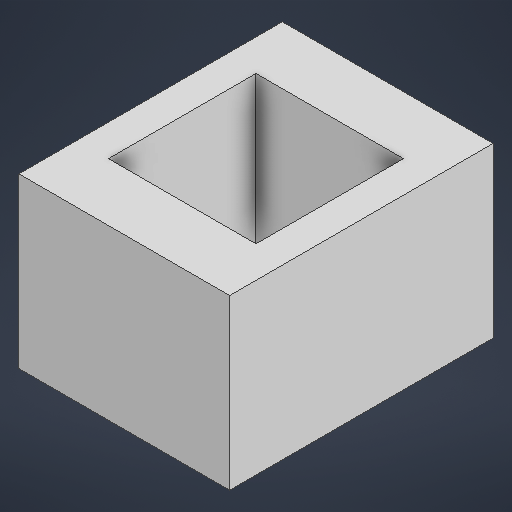
# Autodesk Inventor part: Double Slit Centre Piece
Saved by Autodesk Inventor 2026.1 (Build 301233020, 233B)
## iProperties
Created: 2026-02-12
Part Number: Double Slit Centre Piece
Material: Generic
Document SubType Name: Modeling
Designer: jacob
Density: 1 g/cm^3
Appearance: Default
Author: jacob
Autodesk Inventor part; units mm, degrees
ref_plane "YZ Plane" through (0, 0, 0) normal (1, 0, 0) x (0, 1, 0)
ref_plane "XZ Plane" through (0, 0, 0) normal (0, 1, 0) x (-1, 0, 0)
ref_plane "XY Plane" through (0, 0, 0) normal (0, 0, 1) x (1, 0, 0)
sketch "Sketch1" plane through (0, 0, 0) normal (0, 1, 0) x (-1, 0, 0)
  line L0 (2.5, 3.125) -> (-2.5, 3.125)
  line L1 (-2.5, 3.125) -> (-2.5, -3.125)
  line L2 (-2.5, -3.125) -> (2.5, -3.125)
  line L3 (2.5, -3.125) -> (2.5, 3.125)
  dimension "d3" = 5
  constraints: 8 end point, 2 perpendicular, 1 vertical
  measures "d3" distance of L0.start L0.end
extrude "Extrusion1" add sketch "Sketch1" along normal blind 4
sketch "Sketch2" plane through (0, 4, 0) normal (0, 1, 0) x (1, 0, 0)
  line L0 (-1.75, -1.75) -> (1.75, -1.75)
  line L1 (1.75, -1.75) -> (1.75, 1.75)
  line L2 (1.75, 1.75) -> (-1.75, 1.75)
  line L3 (-1.75, 1.75) -> (-1.75, -1.75)
  dimension "d9" = 3.5
  constraints: 8 end point, 3 perpendicular
  measures "d9" distance of L0.start L0.end
extrude "Extrusion2" cut sketch "Sketch2" against normal blind 3.5
body "Solid1"
